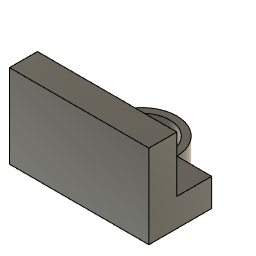
EX-03 (Autodesk Fusion 360 design; units mm, degrees)
Autodesk Fusion 360 part; units mm, degrees
sketch "Sketch1" plane through (0, 0, 0) normal (0, 0, 1) x (1, 0, 0)
sketch "Sketch2" plane through (0, 0, 0) normal (0, 1, 0) x (1, 0, 0)
  line L0 (0, 0) -> (100, 0)
  line L1 (100, 0) -> (100, -60)
  line L2 (100, -60) -> (0, -60)
  line L3 (0, -60) -> (0, 0)
  dimension "d1" = 100
  dimension "d2" = 60
  constraint horizontal L0
  constraint vertical L1
  constraint horizontal L2
  constraint vertical L3
  constraint coincident L0.start L3.end
  measures "d1" distance of L0.start L0.end
  measures "d2" distance of L0.start L2.end
extrude "Extrude1" add sketch "Sketch2" along normal blind 20
sketch "Sketch3" plane through (0, 20, 0) normal (0, 1, 0) x (-1, 0, 0)
  line L0 (0, 60) -> (-100, 60)
  line L1 (-100, 60) -> (-100, 0)
  line L2 (-100, 0) -> (0, 0)
  line L3 (0, 0) -> (0, 60)
  line L4 (0, 20) -> (-100, 20)
  dimension "d5" = 20
  constraint coincident L3 L4.start
  constraint coincident L1 L4.end
  constraint perpendicular L1 L4
  measures "d5" distance of L2 L4
extrude "Extrude2" add sketch "Sketch3" along normal blind 50 contours L1 L2 L3 L4
sketch "Sketch4" plane through (0, 0, 20) normal (0, 0, 1) x (-1, 0, 0)
  line L0 (0, -20) -> (-100, -20)
  line L1 (-100, -20) -> (-100, -70)
  line L2 (-100, -70) -> (0, -70)
  line L3 (0, -70) -> (0, -20)
  circle A0 centre (-50, -45) radius 20
  circle A1 centre (-50, -45) radius 25
  line L4 (0, -45) -> (-25, -45)
  line L5 (-75, -45) -> (-100, -45)
  dimension "d8" = 40
  dimension "d9" = 50
  constraint concentric A0 A1
  constraint midpoint L3 L4.start
  constraint coincident A1 L4.end
  constraint perpendicular L3 L4
  constraint coincident A1 L5.start
  constraint midpoint L1 L5.end
  constraint perpendicular L1 L5
  measures "d8" diameter of A0
  measures "d9" diameter of A1
extrude "Extrude3" cut sketch "Sketch4" against normal blind 20 contours L2 L3 A1 L4 | L1 L2 A1 L5 | A0
